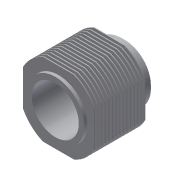
# Autodesk Inventor part: Rcylinder
Saved by Autodesk Inventor 2022 Beta2 (Build 260130000, 130) ContinuousBuild 0
## iProperties
Shininess: 64.0
Angle Display Precision: 2
Document Length Units: 11272
Document Angle Units: 11279
Document Time Units: 11290
Document Mass Units: 11286
Document Length Units Precision: 3
Document Angle Units Precision: 2
Created: 2002-04-22
Part Number: Rcylinder
Material: Aluminum-6061
Document SubType Name: Modeling
Designer: Nino
Density: 2.71 g/cm^3
Appearance: Aluminum - Flat-1
Density: 0.0
Volumn: 0.0
Area: 0.0
PropertySet Name: Model Information
Control State: 0
Master: False
Checked Out: False
Author: Nino
Autodesk Inventor part; units mm, degrees
sketch "Sketch1" plane through (0, 0, 0) normal (0, 0, 1) x (1, 0, 0)
  circle A0 centre (106.1115, 93.472) radius 92.202 projected
  circle A1 centre (106.1115, 93.472) radius 101.346
  dimension "d2" = 9.144
  constraints: 1 centre point
  measures "d2" radial gap between concentric circles of A1 A0
extrude "Extrusion1" add sketch "Sketch1" against normal blind 6.35
sketch "Sketch2" plane through (106.1115, 93.472, 0) normal (0, 0, 1) x (1, 0, 0)
  circle A0 centre (0, 0) radius 92.202 projected
  circle A1 centre (0, 0) radius 101.346 projected
  circle A2 centre (0, 0) radius 82.55
  dimension "d5" = 9.652
  constraints: 1 centre point
  measures "d5" radial gap between concentric circles of A0 A2
extrude "Extrusion2" add sketch "Sketch2" along normal blind 228.6 contours A0 | A1
extrude "Extrusion3" add sketch "Sketch2" against normal blind 15.24 contours A0
ref_plane "Work Plane1" through (106.1115, 93.472, 38.1) normal (0, 0, -1) x (-1, 0, 0)
sketch "Sketch3" plane through (106.1115, 93.472, 38.1) normal (0, 0, -1) x (-1, 0, 0)
  circle A0 centre (0, 0) radius 101.346 projected
  line L0 (-124.7192, 63.5) -> (-124.7192, -63.5)
  line L1 (-53.475, 129.335) -> (53.475, 129.335)
  line L2 (-54.6117, -128.8592) -> (54.6117, -128.8592)
  line L3 (124.7192, 63.5) -> (124.7192, -63.5)
  arc A1 (-53.475, 129.335) -> (-124.7192, 63.5) centre (0, 0) ccw
  arc A2 (-124.7192, -63.5) -> (-54.6117, -128.8592) centre (0, 0) ccw
  arc A3 (54.6117, -128.8592) -> (124.7192, -63.5) centre (0, 0) ccw
  arc A4 (124.7192, 63.5) -> (53.475, 129.335) centre (0, 0) ccw
  dimension "d12" = 63.5
  dimension "d13" = 63.5
  dimension "d14" = 54.6117
  dimension "d15" = 53.475
  constraints: 8 end point, 8 point on circle, 4 centre point, 2 perpendicular, 1 parallel, 1 vertical
  measures "d12" vertical distance of A0.centre L0.start
  measures "d13" vertical distance of A0.centre L3.start
  measures "d14" horizontal distance of A0.centre L2.start
  measures "d15" horizontal distance of A0.centre L1.start
extrude "Extrusion4" add sketch "Sketch3" along normal mid plane 3.175
pattern_linear "Rectangular Pattern1" count 15 spacing 12.7 along (0, 0, 1) of "Extrusion4"
ref_plane "Work Plane2" through (106.1115, 93.472, 0) normal (0, 1, 0) x (0, 0, 1)
ref_plane "Work Plane3" through (106.1115, 93.472, 0) normal (1, 0, 0) x (0, 0, 1)
equation "\"d13\" = d12"
body "Solid1"
